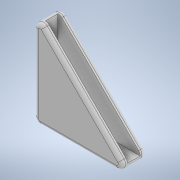
# Autodesk Inventor part: Mirror Corner
Saved by Autodesk Inventor 2021.2 (Build 252289000, 289)
## iProperties
Created: 2021-02-09
Part Number: Mirror Corner
Material: Generic
Document SubType Name: Modeling
Designer: robst
Density: 1 g/cm^3
Appearance: Default
Author: robst
Autodesk Inventor part; units mm, degrees
ref_plane "YZ Plane" through (0, 0, 0) normal (1, 0, 0) x (0, 1, 0)
ref_plane "XZ Plane" through (0, 0, 0) normal (0, 1, 0) x (-1, 0, 0)
ref_plane "XY Plane" through (0, 0, 0) normal (0, 0, 1) x (1, 0, 0)
sketch "Sketch1" plane through (0, 0, 0) normal (0, 0, 1) x (1, 0, 0)
  line L0 (0, 0) -> (-13.377, 0)
  line L1 (0, 0) -> (0, 26.67)
  line L2 (0, 26.67) -> (26.67, 0)
  line L3 (26.67, 0) -> (0, 0)
  dimension "d0" = 26.67
  constraints: 8 end point, 2 perpendicular, 1 horizontal, 1 vertical
  measures "d0" distance of L0.start L1.end
extrude "Extrusion1" add sketch "Sketch1" along normal mid plane 6.604
sketch "Sketch3" plane through (0, 0, 0) normal (0, 0, 1) x (1, 0, 0)
  line L0 (0, 26.67) -> (26.67, 0) projected
  line L1 (0, 0) -> (0, 26.67) projected
  line L2 (26.67, 0) -> (0, 0) projected
  line L3 (1.524, 25.146) -> (1.524, 1.524)
  line L4 (1.524, 1.524) -> (25.146, 1.524)
  line L5 (1.524, 25.146) -> (25.146, 1.524)
  dimension "d3" = 1.524
  dimension "d4" = 1.524
  constraints: 6 end point, 2 point on line, 1 collinear, 1 horizontal, 1 vertical
  measures "d3" distance between parallel lines of L3 L1
  measures "d4" distance between parallel lines of L4 L2
extrude "Extrusion2" cut sketch "Sketch3" against normal mid plane 3.556 contours L0 L4 L3
fillet "Fillet1" radius 1.524 3 edges at (0, 26.67, 0) (0, 0, 0) (26.67, 0, 0)
fillet "Fillet2" radius 1.016 6 edges at (0.4464, 0.4464, 3.302) (12.2574, 0, 3.302) (24.3987, 0.9408, 3.302) (13.335, 13.335, 3.302) (0.9408, 24.3987, 3.302) (0, 12.2574, 3.302)
fillet "Fillet3" radius 1.016 6 edges at (0.9408, 24.3987, -3.302) (13.335, 13.335, -3.302) (24.3987, 0.9408, -3.302) (12.2574, 0, -3.302) (0.4464, 0.4464, -3.302) (0, 12.2574, -3.302)
equation "\"d0\" = edgeSize"
equation "\"d1\" = partThickness"
equation "\"d3\" = edgeThickness"
equation "\"d4\" = edgeThickness"
equation "\"d5\" = mirrorThickness"
equation "\"d7\" = filetForCorners"
equation "\"d8\" = filetForFlat"
equation "\"d9\" = filetForFlat"
equation "\"edgeSize\" = 26.67"
equation "\"wallThickness\" = 1.524"
equation "\"mirrorThickness\" = 3.556"
equation "\"partThickness\" = mirrorThickness + 2 * wallThickness"
equation "\"edgeThickness\" = 1.524"
equation "\"filetForCorners\" = 1.524"
equation "\"filetForFlat\" = 1.016"
body "Solid1"
